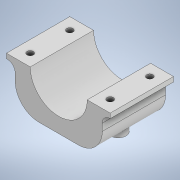
# Autodesk Inventor part: mocowanie silnika dolne
Saved by Autodesk Inventor 2021 (Build 250183000, 183)
## iProperties
Created: 2021-06-29
Part Number: mocowanie silnika dolne
Material: Generic
Document SubType Name: Modeling
Designer: Łukasz
Density: 1 g/cm^3
Appearance: Default
Author: Łukasz
Autodesk Inventor part; units mm, degrees
ref_plane "YZ Plane" through (0, 0, 0) normal (1, 0, 0) x (0, 1, 0)
ref_plane "XZ Plane" through (0, 0, 0) normal (0, 1, 0) x (-1, 0, 0)
ref_plane "XY Plane" through (0, 0, 0) normal (0, 0, 1) x (1, 0, 0)
sketch "Sketch1" plane through (0, 0, 0) normal (0, 0, 1) x (1, 0, 0)
  arc A0 (-18, 0) -> (18, 0) centre (0, 0) ccw
  arc A1 (0, -27.5) -> (27.5, 0) centre (0, 0) ccw construction
  line L0 (27.5, -8) -> (27.5, -12.5)
  line L1 (12.5, -27.5) -> (-12.5, -27.5)
  line L2 (-27.5, -12.5) -> (-27.5, -8)
  line L3 (-27.5, 0) -> (-18, 0)
  line L4 (18, 0) -> (27.5, 0)
  line L5 (-18, 0) -> (-33, 0)
  line L6 (-33, 0) -> (-33, -3)
  line L7 (-33, -3) -> (-32.5, -3)
  arc A2 (-27.5, -8) -> (-32.5, -3) centre (-32.5, -8) ccw
  line L8 (27.5, 0) -> (32.5, 0)
  line L9 (32.5, 0) -> (32.5, -3)
  line L10 (32.5, -3) -> (32.5, -3)
  arc A3 (32.5, -3) -> (27.5, -8) centre (32.5, -8) ccw
  arc A4 (-27.5, -12.5) -> (-12.5, -27.5) centre (-12.5, -12.5) ccw
  arc A5 (12.5, -27.5) -> (27.5, -12.5) centre (12.5, -12.5) ccw
  point P0 (27.5, -27.5)
  point P1 (-27.5, -27.5)
  dimension "d0" = 36
  dimension "d1" = 55
  dimension "d2" = 15
  dimension "d3" = 3
  dimension "d4" = 5
  dimension "d5" = 5
  dimension "d6" = 3
  dimension "d7" = 90
  dimension "d8" = 5
  dimension "d11" = 15
  constraints: 22 end point, 12 point on circle, 8 tangent, 7 point on line, 6 centre point, 4 perpendicular, 3 horizontal, 3 parallel, 2 coincident, 1 equal radius, 1 midpoint, 1 vertical
  measures "d0" diameter of A0
  measures "d1" diameter of A1
  measures "d2" distance of L3.end L5.end
  measures "d3" distance of L5.end L6.end
  measures "d4" radius of A2
  measures "d5" distance of L4.end L8.end
  measures "d6" distance of L8.end L9.end
  measures "d7" angle of L9 L10
  measures "d8" radius of A3
  measures "d11" radius of A4
extrude "Extrusion1" add sketch "Sketch1" along normal blind 40
sketch "Sketch2" plane through (-12.5, -27.5, 0) normal (0, -1, 0) x (1, 0, 0)
  circle A0 centre (-5, 20) radius 5
  circle A1 centre (30, 20) radius 5
  line L0 (-5, 25) -> (30.5, 24.9749)
  line L1 (30.5, 0) -> (30.5, 40) projected
  line L2 (30.5, 15.0251) -> (-5.5, 15.0251)
  line L3 (-5.5, 0) -> (-5.5, 40) projected
  point P0 (12.5, 0)
  dimension "d12" = 10
  dimension "d13" = 10
  constraints: 4 end point, 4 point on circle, 3 point on line, 2 centre point
  measures "d12" diameter of A0
  measures "d13" diameter of A1
extrude "Extrusion2" add sketch "Sketch2" against normal blind 5 contours A0 L2 L3 | A0 L0 A1 L2 | L3 A0 | L0 L1 L2 A1 | A1 L1
sketch "Sketch3" plane through (-12.5, -27.5, 0) normal (0, -1, 0) x (1, 0, 0)
  arc A0 (-5, 25) -> (-5.5, 15.0251) centre (-5, 20) ccw projected
  circle A1 centre (-5, 20) radius 2
  arc A2 (30.5, 15.0251) -> (30.5, 24.9749) centre (30, 20) ccw projected
  circle A3 centre (30, 20) radius 2
  point P0 (12.5, 0)
  dimension "d16" = 4
  dimension "d17" = 4
  constraints: 2 centre point, 2 coincident
  measures "d16" diameter of A1
  measures "d17" diameter of A3
extrude "Extrusion3" cut sketch "Sketch3" against normal blind 15
sketch "Sketch4" plane through (18, 0, 0) normal (0, 1, 0) x (1, 0, 0)
  circle A0 centre (-43.5, -32.5) radius 2
  line L0 (-36, -40) -> (-51, -40) projected
  line L1 (-51, 0) -> (-51, -40) projected
  circle A1 centre (7, -32.5) radius 2
  circle A2 centre (-43.5, -7.5) radius 2
  circle A3 centre (7, -7.5) radius 2
  point P0 (-18, 0)
  dimension "d20" = 4
  dimension "d21" = 7.5
  dimension "d22" = 7.5
  dimension "d25" = 50.5
  dimension "d28" = 25
  constraints: 4 centre point, 1 horizontal, 1 vertical, 6 other
  measures "d20" diameter of A0
  measures "d21" distance from line of L0 A0.centre
  measures "d22" distance from line of L1 A0.centre
  measures "d25" distance of A0.centre A1.centre
  measures "d28" distance of A0.centre A2.centre
extrude "Extrusion4" cut sketch "Sketch4" against normal blind 10
body "Solid1"
